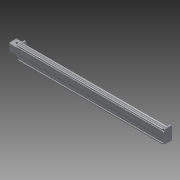
# Autodesk Inventor part: GL15N21240NSW' Body2
Saved by Autodesk Inventor 2011 SP1 (Build 150282100, 282)
## iProperties
Created: 2013-10-23
Part Number: GL15N21240NSW' Body2
Catalog Web Link: www.cadenas.de
Description: Type GL-N-body2-
Vendor: THK
Document SubType Name: Modeling
Designer: PARTuser1
Manufacturer: THK
Density: 1 g/cm^3
Category: PARTsolutions
Company: THK
Title: GL15N21240NSW' Body2
Author: Cadenas PARTsolutions
PSOL_IDENT_0: {$CADENAS_DATA\23d-libs\thk\actuator\type_gl_n\type_gl_n_f_na_1.prj},213 {VTYP=3D},{NB=GL15N21240NSW
PSOL_IDENT_1: ' Body2},{LINA=GL15N21240NSW' Body2},{NN=Type GL-N-body2},{DATE=29.11.2012 11:43:39},{GEOMDATE=29.11
PSOL_IDENT_2: .2012 11:43:00},{VERSION=},{LINEID=20},{LINESUBID=-1},{WBVAR=L,C,LM,BSE,BSM,LML,BSL}  {NB=GL15N21240
PSOL_IDENT_3: NSW' Body2},{LINA=GL15N21240NSW' Body2},{KT=DUMMY},{IDNR=},{MN=GL15N},{L=1240},{C=N},{LX=340,460,580
PSOL_IDENT_4: ,700,820,1060,1240,1420,1600,1780,1960},{LM=SW},{VER=2},{DS=Belt kit},{BSE=},{R=25.000},{NDM=2.000},
PSOL_IDENT_5: {PCD=0.000},{BSM=},{BSE1='','None'},{SD=39},{SD1=27},{TL=154.000},{B=52.000},{TL1=180.000},{B1=55.00
PSOL_IDENT_6: 0},{DS1=Ex},{LML='},{BSL=},{BSL1='','None'},{N=7},{N1=5},{N2=7.000},{N3=5},{BSM1='','None'}
CNS_NB: GL15N21240NSW' Body2
CNS_NBSYN: $MN.$VER.$L.$C.$BSE.$BSM.$LM.$LML.$BSL. Body2
CNS_LINA: GL15N21240NSW' Body2
CNS_MN: GL15N
CNS_L: 1240
CNS_C: No
CNS_LX: 340,460,580,700,820,1060,1240,1420,1600,1780,1960
CNS_LM: SSR-XW (L-type table)
CNS_VER: 2
CNS_DS: Belt kit
CNS_R: 25.000
CNS_NDM: 2.000
CNS_PCD: 0.000
CNS_BSE1: '','None'
CNS_SD: 39
CNS_SD1: 27
CNS_TL: 154.000
CNS_B: 52.000
CNS_TL1: 180.000
CNS_B1: 55.000
CNS_DS1: Ex
CNS_LML: No mark:Not provided with QZ
CNS_BSL1: '','None'
CNS_N: 7.000
CNS_N1: 5.000
CNS_N2: 7.000
CNS_N3: 5.000
CNS_BSM1: '','None'
SUPPLIER: THK
ARTICLENO: GL15N21240NSW' Body2
BOMINFO: GL15N21240NSW' Body2
CREATOR: CADENAS GmbH
Autodesk Inventor part; units mm, degrees
sketch "Sketch_1" plane through (0, 0, 0) normal (1, 0, 0) x (0, 1, 0)
  line L0 (18.1, 58) -> (12.47, 58)
  arc A0 (12.47, 58) -> (12, 57.53) centre (12.47, 57.53) ccw
  line L1 (12, 57.53) -> (12, 54.97)
  arc A1 (11.53, 54.5) -> (12, 54.97) centre (11.53, 54.97) ccw
  line L2 (11.53, 54.5) -> (6.47, 54.5)
  arc A2 (6, 54.97) -> (6.47, 54.5) centre (6.47, 54.97) ccw
  line L3 (6, 54.97) -> (6, 57.53)
  arc A3 (6, 57.53) -> (5.53, 58) centre (5.53, 57.53) ccw
  line L4 (5.53, 58) -> (3.14, 58)
  arc A4 (3.14, 58) -> (0, 54.86) centre (3.14, 54.86) ccw
  line L5 (0, 54.86) -> (0, 48.5)
  arc A5 (0, 48.5) -> (0.5, 48) centre (0.5, 48.5) ccw
  line L6 (0.5, 48) -> (3.5, 48)
  arc A6 (3.5, 48) -> (4, 48.5) centre (3.5, 48.5) ccw
  line L7 (4, 48.5) -> (4, 50)
  arc A7 (4.5, 50.5) -> (4, 50) centre (4.5, 50) ccw
  line L8 (4.5, 50.5) -> (8.5, 50.5)
  arc A8 (9, 50) -> (8.5, 50.5) centre (8.5, 50) ccw
  line L9 (9, 50) -> (9, 48.8)
  arc A9 (9, 48.8) -> (9.3, 48.5) centre (9.3, 48.8) ccw
  line L10 (9.3, 48.5) -> (9.7, 48.5)
  arc A10 (10, 48.2) -> (9.7, 48.5) centre (9.7, 48.2) ccw
  line L11 (10, 48.2) -> (10, 41.8)
  arc A11 (9.7, 41.5) -> (10, 41.8) centre (9.7, 41.8) ccw
  line L12 (9.7, 41.5) -> (9.3, 41.5)
  arc A12 (9.3, 41.5) -> (9, 41.2) centre (9.3, 41.2) ccw
  line L13 (9, 41.2) -> (9, 40)
  arc A13 (8.5, 39.5) -> (9, 40) centre (8.5, 40) ccw
  line L14 (8.5, 39.5) -> (4.5, 39.5)
  arc A14 (4, 40) -> (4.5, 39.5) centre (4.5, 40) ccw
  line L15 (4, 40) -> (4, 41.5)
  arc A15 (4, 41.5) -> (3.5, 42) centre (3.5, 41.5) ccw
  line L16 (3.5, 42) -> (0.5, 42)
  arc A16 (0.5, 42) -> (0, 41.5) centre (0.5, 41.5) ccw
  line L17 (0, 41.5) -> (0, 24)
  line L18 (0, 24) -> (0.531, 22.938)
  arc A17 (0.635, 22.4347) -> (0.531, 22.938) centre (-0.3634, 22.4908) ccw
  arc A18 (0.635, 22.4347) -> (0.635, -22.4347) centre (400.0054, 0) ccw
  arc A19 (0.531, -22.938) -> (0.635, -22.4347) centre (-0.3634, -22.4908) ccw
  line L19 (0.531, -22.938) -> (0, -24)
  line L20 (0, -24) -> (0, -41.5)
  arc A20 (0, -41.5) -> (0.5, -42) centre (0.5, -41.5) ccw
  line L21 (0.5, -42) -> (3.5, -42)
  arc A21 (3.5, -42) -> (4, -41.5) centre (3.5, -41.5) ccw
  line L22 (4, -41.5) -> (4, -40)
  arc A22 (4.5, -39.5) -> (4, -40) centre (4.5, -40) ccw
  line L23 (4.5, -39.5) -> (8.5, -39.5)
  arc A23 (9, -40) -> (8.5, -39.5) centre (8.5, -40) ccw
  line L24 (9, -40) -> (9, -41.2)
  arc A24 (9, -41.2) -> (9.3, -41.5) centre (9.3, -41.2) ccw
  line L25 (9.3, -41.5) -> (9.7, -41.5)
  arc A25 (10, -41.8) -> (9.7, -41.5) centre (9.7, -41.8) ccw
  line L26 (10, -41.8) -> (10, -48.2)
  arc A26 (9.7, -48.5) -> (10, -48.2) centre (9.7, -48.2) ccw
  line L27 (9.7, -48.5) -> (9.3, -48.5)
  arc A27 (9.3, -48.5) -> (9, -48.8) centre (9.3, -48.8) ccw
  line L28 (9, -48.8) -> (9, -50)
  arc A28 (8.5, -50.5) -> (9, -50) centre (8.5, -50) ccw
  line L29 (8.5, -50.5) -> (4.5, -50.5)
  arc A29 (4, -50) -> (4.5, -50.5) centre (4.5, -50) ccw
  line L30 (4, -50) -> (4, -48.5)
  arc A30 (4, -48.5) -> (3.5, -48) centre (3.5, -48.5) ccw
  line L31 (3.5, -48) -> (0.5, -48)
  arc A31 (0.5, -48) -> (0, -48.5) centre (0.5, -48.5) ccw
  line L32 (0, -48.5) -> (0, -54.86)
  arc A32 (0, -54.86) -> (3.14, -58) centre (3.14, -54.86) ccw
  line L33 (3.14, -58) -> (5.53, -58)
  arc A33 (5.53, -58) -> (6, -57.53) centre (5.53, -57.53) ccw
  line L34 (6, -57.53) -> (6, -54.97)
  arc A34 (6.47, -54.5) -> (6, -54.97) centre (6.47, -54.97) ccw
  line L35 (6.47, -54.5) -> (11.53, -54.5)
  arc A35 (12, -54.97) -> (11.53, -54.5) centre (11.53, -54.97) ccw
  line L36 (12, -54.97) -> (12, -57.53)
  arc A36 (12, -57.53) -> (12.47, -58) centre (12.47, -57.53) ccw
  line L37 (12.47, -58) -> (18.1, -58)
  line L38 (18.1, -58) -> (18.1, -57)
  line L39 (18.1, -57) -> (20.98, -57)
  arc A37 (20.98, -57) -> (21.45, -56.53) centre (20.98, -56.53) ccw
  line L40 (21.45, -56.53) -> (21.45, -55.97)
  arc A38 (21.45, -55.97) -> (20.98, -55.5) centre (20.98, -55.97) ccw
  line L41 (20.98, -55.5) -> (20.9, -55.5)
  arc A39 (20.7, -55.3) -> (20.9, -55.5) centre (20.9, -55.3) ccw
  line L42 (20.7, -55.3) -> (20.7, -53.3)
  arc A40 (21, -53) -> (20.7, -53.3) centre (21, -53.3) ccw
  line L43 (21, -53) -> (22, -53)
  arc A41 (22, -53) -> (22.2, -52.8) centre (22, -52.8) ccw
  arc A42 (22.5, -52.5) -> (22.2, -52.8) centre (22.5, -52.8) ccw
  line L44 (22.5, -52.5) -> (24.7, -52.5)
  arc A43 (25, -52.8) -> (24.7, -52.5) centre (24.7, -52.8) ccw
  arc A44 (25, -52.8) -> (25.2, -53) centre (25.2, -52.8) ccw
  line L45 (25.2, -53) -> (26.2, -53)
  arc A45 (26.5, -53.3) -> (26.2, -53) centre (26.2, -53.3) ccw
  line L46 (26.5, -53.3) -> (26.5, -55.3)
  arc A46 (26.3, -55.5) -> (26.5, -55.3) centre (26.3, -55.3) ccw
  line L47 (26.3, -55.5) -> (26.22, -55.5)
  arc A47 (26.22, -55.5) -> (25.75, -55.97) centre (26.22, -55.97) ccw
  line L48 (25.75, -55.97) -> (25.75, -56.53)
  arc A48 (25.75, -56.53) -> (26.22, -57) centre (26.22, -56.53) ccw
  line L49 (26.22, -57) -> (29.1, -57)
  line L50 (29.1, -57) -> (29.1, -58)
  line L51 (29.1, -58) -> (31.6, -58)
  line L52 (31.6, -58) -> (33, -56.6)
  line L53 (33, -56.6) -> (33, -52.5)
  line L54 (33, -52.5) -> (34.32, -52.5)
  line L55 (34.32, -52.5) -> (37.42, -49.4)
  line L56 (37.42, -49.4) -> (40.4, -49.4)
  line L57 (40.4, -49.4) -> (43.5, -52.5)
  line L58 (43.5, -52.5) -> (44.8, -52.5)
  line L59 (44.8, -52.5) -> (45.6, -51.7)
  line L60 (45.6, -51.7) -> (45.6, -38.3)
  line L61 (45.6, -38.3) -> (44.8, -37.5)
  line L62 (44.8, -37.5) -> (43.5, -37.5)
  line L63 (43.5, -37.5) -> (40.37, -40.63)
  line L64 (40.37, -40.63) -> (37.45, -40.63)
  line L65 (37.45, -40.63) -> (34.32, -37.5)
  line L66 (34.32, -37.5) -> (32.2, -37.5)
  line L67 (32.2, -37.5) -> (32.2, -33.5)
  arc A49 (32.2, -33.5) -> (31.7, -33) centre (31.7, -33.5) ccw
  line L68 (31.7, -33) -> (17, -33)
  arc A50 (16, -32) -> (17, -33) centre (17, -32) ccw
  line L69 (16, -32) -> (16, 32)
  arc A51 (17, 33) -> (16, 32) centre (17, 32) ccw
  line L70 (17, 33) -> (31.7, 33)
  arc A52 (31.7, 33) -> (32.2, 33.5) centre (31.7, 33.5) ccw
  line L71 (32.2, 33.5) -> (32.2, 37.5)
  line L72 (32.2, 37.5) -> (34.32, 37.5)
  line L73 (34.32, 37.5) -> (37.45, 40.63)
  line L74 (37.45, 40.63) -> (40.37, 40.63)
  line L75 (40.37, 40.63) -> (43.5, 37.5)
  line L76 (43.5, 37.5) -> (44.8, 37.5)
  line L77 (44.8, 37.5) -> (45.6, 38.3)
  line L78 (45.6, 38.3) -> (45.6, 51.7)
  line L79 (45.6, 51.7) -> (44.8, 52.5)
  line L80 (44.8, 52.5) -> (43.5, 52.5)
  line L81 (43.5, 52.5) -> (40.4, 49.4)
  line L82 (40.4, 49.4) -> (37.42, 49.4)
  line L83 (37.42, 49.4) -> (34.32, 52.5)
  line L84 (34.32, 52.5) -> (33, 52.5)
  line L85 (33, 52.5) -> (33, 56.6)
  line L86 (33, 56.6) -> (31.6, 58)
  line L87 (31.6, 58) -> (29.1, 58)
  line L88 (29.1, 58) -> (29.1, 57)
  line L89 (29.1, 57) -> (26.22, 57)
  arc A53 (26.22, 57) -> (25.75, 56.53) centre (26.22, 56.53) ccw
  line L90 (25.75, 56.53) -> (25.75, 55.97)
  arc A54 (25.75, 55.97) -> (26.22, 55.5) centre (26.22, 55.97) ccw
  line L91 (26.22, 55.5) -> (26.3, 55.5)
  arc A55 (26.5, 55.3) -> (26.3, 55.5) centre (26.3, 55.3) ccw
  line L92 (26.5, 55.3) -> (26.5, 53.3)
  arc A56 (26.2, 53) -> (26.5, 53.3) centre (26.2, 53.3) ccw
  line L93 (26.2, 53) -> (25.2, 53)
  arc A57 (25.2, 53) -> (25, 52.8) centre (25.2, 52.8) ccw
  arc A58 (24.7, 52.5) -> (25, 52.8) centre (24.7, 52.8) ccw
  line L94 (24.7, 52.5) -> (22.5, 52.5)
  arc A59 (22.2, 52.8) -> (22.5, 52.5) centre (22.5, 52.8) ccw
  arc A60 (22.2, 52.8) -> (22, 53) centre (22, 52.8) ccw
  line L95 (22, 53) -> (21, 53)
  arc A61 (20.7, 53.3) -> (21, 53) centre (21, 53.3) ccw
  line L96 (20.7, 53.3) -> (20.7, 55.3)
  arc A62 (20.9, 55.5) -> (20.7, 55.3) centre (20.9, 55.3) ccw
  line L97 (20.9, 55.5) -> (20.98, 55.5)
  arc A63 (20.98, 55.5) -> (21.45, 55.97) centre (20.98, 55.97) ccw
  line L98 (21.45, 55.97) -> (21.45, 56.53)
  arc A64 (21.45, 56.53) -> (20.98, 57) centre (20.98, 56.53) ccw
  line L99 (20.98, 57) -> (18.1, 57)
  line L100 (18.1, 57) -> (18.1, 58)
  constraints: 202 end point, 130 point on circle, 65 centre point
extrude "Extrusion1" add sketch "Sketch_1" along normal blind 1240
sketch "Sketch_2" plane through (0, 0, 0) normal (1, 0, 0) x (0, 1, 0)
  line L0 (68.3, 57) -> (27.6, 57)
  line L1 (27.6, 57) -> (27.6, 53)
  line L2 (27.6, 53) -> (19.6, 53)
  line L3 (19.6, 53) -> (19.6, 57)
  line L4 (19.6, 57) -> (12.12, 57)
  line L5 (12.12, 57) -> (10, 54.88)
  line L6 (10, 54.88) -> (10, 38.5)
  line L7 (10, 38.5) -> (3.41, 38.5)
  line L8 (3.41, 38.5) -> (2, 37.09)
  line L9 (2, 37.09) -> (2, -37.09)
  line L10 (2, -37.09) -> (3.41, -38.5)
  line L11 (3.41, -38.5) -> (10, -38.5)
  line L12 (10, -38.5) -> (10, -54.88)
  line L13 (10, -54.88) -> (12.12, -57)
  line L14 (12.12, -57) -> (19.6, -57)
  line L15 (19.6, -57) -> (19.6, -53)
  line L16 (19.6, -53) -> (27.6, -53)
  line L17 (27.6, -53) -> (27.6, -57)
  line L18 (27.6, -57) -> (68.3, -57)
  line L19 (68.3, -57) -> (68.3, -50)
  line L20 (68.3, -50) -> (72.3, -50)
  line L21 (72.3, -50) -> (72.3, 50)
  line L22 (72.3, 50) -> (68.3, 50)
  line L23 (68.3, 50) -> (68.3, 57)
  constraints: 48 end point
extrude "Extrusion2" add sketch "Sketch_2" against normal blind 12
sketch "Sketch_3" plane through (1240, 0, 0) normal (1, 0, 0) x (0, 0, -1)
  line L0 (-57, 68.3) -> (-57, 27.6)
  line L1 (-57, 27.6) -> (-53, 27.6)
  line L2 (-53, 27.6) -> (-53, 19.6)
  line L3 (-53, 19.6) -> (-57, 19.6)
  line L4 (-57, 19.6) -> (-57, 12.12)
  line L5 (-57, 12.12) -> (-54.88, 10)
  line L6 (-54.88, 10) -> (-38.5, 10)
  line L7 (-38.5, 10) -> (-38.5, 3.41)
  line L8 (-38.5, 3.41) -> (-37.09, 2)
  line L9 (-37.09, 2) -> (37.09, 2)
  line L10 (37.09, 2) -> (38.5, 3.41)
  line L11 (38.5, 3.41) -> (38.5, 10)
  line L12 (38.5, 10) -> (54.88, 10)
  line L13 (54.88, 10) -> (57, 12.12)
  line L14 (57, 12.12) -> (57, 19.6)
  line L15 (57, 19.6) -> (53, 19.6)
  line L16 (53, 19.6) -> (53, 27.6)
  line L17 (53, 27.6) -> (57, 27.6)
  line L18 (57, 27.6) -> (57, 68.3)
  line L19 (57, 68.3) -> (50, 68.3)
  line L20 (50, 68.3) -> (50, 72.3)
  line L21 (50, 72.3) -> (-50, 72.3)
  line L22 (-50, 72.3) -> (-50, 68.3)
  line L23 (-50, 68.3) -> (-57, 68.3)
  constraints: 48 end point
extrude "Extrusion3" add sketch "Sketch_3" along normal blind 12
sketch "Sketch4" plane through (0, 72.3, 50) normal (0, 1, 0) x (1, 0, 0)
  point P0 (-6, 82)
hole "Drilling 1" at (-6, 72.3, -32) direction (0, -1, 0) diameter 2.459 depth 5.5 tip angle 120.691 countersink diameter 3 countersink angle 90 thread size "M3x0.5" class "6H" standard "ISO Metric profile"
sketch "Sketch5" plane through (0, 72.3, 50) normal (0, 1, 0) x (1, 0, 0)
  point P0 (-6, 18)
hole "Drilling 2" at (-6, 72.3, 32) direction (0, -1, 0) diameter 2.459 depth 5.5 tip angle 120.691 countersink diameter 3 countersink angle 90 thread size "M3x0.5" class "6H" standard "ISO Metric profile"
sketch "Sketch6" plane through (1240, 72.3, 50) normal (0, 1, 0) x (1, 0, 0)
  point P0 (6, 82)
hole "Drilling 3" at (1246, 72.3, -32) direction (0, -1, 0) diameter 2.459 depth 5.5 tip angle 120.691 countersink diameter 3 countersink angle 90 thread size "M3x0.5" class "6H" standard "ISO Metric profile"
sketch "Sketch7" plane through (1240, 72.3, 50) normal (0, 1, 0) x (1, 0, 0)
  point P0 (6, 18)
hole "Drilling 4" at (1246, 72.3, 32) direction (0, -1, 0) diameter 2.459 depth 5.5 tip angle 120.691 countersink diameter 3 countersink angle 90 thread size "M3x0.5" class "6H" standard "ISO Metric profile"
sketch "Sketch8" plane through (1252, 0, 0) normal (1, 0, 0) x (0, 0, -1)
  point P0 (38, 64.5)
hole "Drilling 5" at (1252, 64.5, -38) direction (-1, 0, 0) diameter 4.134 depth 12 countersink diameter 5 countersink angle 90 thread size "M5x0.8" class "6H" standard "ISO Metric profile"
sketch "Sketch_5" plane through (0, 0, 0) normal (1, 0, 0) x (0, 1, 0)
  line L0 (66.8094, -34) -> (62.1906, -34)
  line L1 (62.1906, -34) -> (59.8812, -38)
  line L2 (59.8812, -38) -> (62.1906, -42)
  line L3 (62.1906, -42) -> (66.8094, -42)
  line L4 (66.8094, -42) -> (69.1188, -38)
  line L5 (69.1188, -38) -> (66.8094, -34)
  constraints: 12 end point
extrude "Extrusion4" add sketch "Sketch_5" along normal blind 3.2
sketch "Sketch_6" plane through (0, 0, -38) normal (0, 0, 1) x (1, 0, 0)
  line L0 (15, 64.5) -> (3.2, 64.5)
  line L1 (3.2, 64.5) -> (3.2, 67)
  line L2 (3.2, 67) -> (6, 67)
  line L3 (6, 67) -> (6, 70.75)
  line L4 (6, 70.75) -> (15, 70.75)
  line L5 (15, 70.75) -> (15, 64.5)
  line L6 (15, 64.5) -> (3.2, 64.5)
  constraints: 14 end point
revolve "Revolution1" add sketch "Sketch_6" angle 360 about axis through (15, 64.5, -38) along (1, 0, 0)
sketch "Sketch_7" plane through (1237.5, 0, 0) normal (1, 0, 0) x (0, 0, -1)
  line L0 (-29, 16) -> (29, 16)
  line L1 (29, 16) -> (29, 30.5)
  line L2 (29, 30.5) -> (-29, 30.5)
  line L3 (-29, 30.5) -> (-29, 16)
  constraints: 8 end point
extrude "Extrusion5" add sketch "Sketch_7" against normal blind 63
sketch "Sketch_8" plane through (0, 30.5, 0) normal (0, 1, 0) x (1, 0, 0)
  line L0 (1142, -29) -> (1223, -29)
  line L1 (1223, -29) -> (1223, 29)
  line L2 (1223, 29) -> (1142, 29)
  line L3 (1142, 29) -> (1142, 17)
  line L4 (1142, 17) -> (1177, 17)
  line L5 (1177, 17) -> (1177, -17)
  line L6 (1177, -17) -> (1142, -17)
  line L7 (1142, -17) -> (1142, -29)
  arc A0 (1182, -20.4) -> (1182, -25.6) centre (1182, -23) ccw
  line L8 (1182, -25.6) -> (1216, -25.6)
  arc A1 (1216, -25.6) -> (1216, -20.4) centre (1216, -23) ccw
  line L9 (1216, -20.4) -> (1182, -20.4)
  arc A2 (1182, 25.6) -> (1182, 20.4) centre (1182, 23) ccw
  line L10 (1182, 20.4) -> (1216, 20.4)
  arc A3 (1216, 20.4) -> (1216, 25.6) centre (1216, 23) ccw
  line L11 (1216, 25.6) -> (1182, 25.6)
  constraints: 24 end point, 8 point on circle, 4 centre point
extrude "Extrusion6" add sketch "Sketch_8" along normal blind 20
sketch "Sketch_9" plane through (0, 0, 0) normal (0, 0, 1) x (1, 0, 0)
  line L0 (-86, 69.3) -> (-86, 11.7)
  line L1 (-86, 11.7) -> (-81.8, 7.5)
  line L2 (-81.8, 7.5) -> (-12, 7.5)
  line L3 (-12, 7.5) -> (-12, 73.5)
  line L4 (-12, 73.5) -> (-81.8, 73.5)
  line L5 (-81.8, 73.5) -> (-86, 69.3)
  constraints: 12 end point
extrude "Extrusion7" add sketch "Sketch_9" along normal mid plane 60
sketch "Sketch_14" plane through (0, 17.5, 0) normal (0, 1, 0) x (1, 0, 0)
  arc A0 (-49, 20) -> (-49, -20) centre (-49, 0) ccw
  line L0 (-49, -20) -> (0, -20)
  line L1 (0, -20) -> (0, 20)
  line L2 (0, 20) -> (-49, 20)
  constraints: 6 end point, 2 point on circle, 1 centre point
extrude "Extrusion8" cut sketch "Sketch_14" along normal blind 46
sketch "Sketch_15" plane through (1152, 0, 0) normal (1, 0, 0) x (0, 0, -1)
  line L0 (31.15, 40.5) -> (-31.15, 40.5)
  line L1 (-31.15, 40.5) -> (-31.15, 45.5)
  line L2 (-31.15, 45.5) -> (-15.3, 45.5)
  line L3 (-15.3, 45.5) -> (-15.3, 60)
  line L4 (-15.3, 60) -> (-13.8, 60)
  line L5 (-13.8, 60) -> (-13.3, 58.05)
  line L6 (-13.3, 58.05) -> (13.3, 58.05)
  line L7 (13.3, 58.05) -> (13.8, 60)
  line L8 (13.8, 60) -> (15.3, 60)
  line L9 (15.3, 60) -> (15.3, 45.5)
  line L10 (15.3, 45.5) -> (31.15, 45.5)
  line L11 (31.15, 45.5) -> (31.15, 40.5)
  line L12 (31.15, 40.5) -> (-31.15, 40.5)
  constraints: 26 end point
revolve "Revolution2" add sketch "Sketch_15" angle 360 about axis through (1152, 40.5, -31.15) along (0, 0, -1)
sketch "Sketch_16" plane through (0, 0, 30) normal (0, 0, 1) x (1, 0, 0)
  circle A0 centre (-49, 40.5) radius 10
  constraints: 1 centre point
extrude "Extrusion9" cut sketch "Sketch_16" along normal mid plane 5
sketch "Sketch17" plane through (0, 0, -30) normal (0, 0, -1) x (-1, 0, 0)
  point P0 (49, 40.5)
hole "Drilling 7" at (-49, 40.5, -30) direction (0, 0, 1) diameter 20 depth 2.5
sketch "Sketch_18" plane through (-49, 0, 0) normal (1, 0, 0) x (0, 0, -1)
  line L0 (28, 40.5) -> (-42, 40.5)
  line L1 (-42, 40.5) -> (-42, 45)
  line L2 (-42, 45) -> (-41.5, 45.5)
  line L3 (-41.5, 45.5) -> (-15.3, 45.5)
  line L4 (-15.3, 45.5) -> (-15.3, 60)
  line L5 (-15.3, 60) -> (-13.8, 60)
  line L6 (-13.8, 60) -> (-13.3, 58.05)
  line L7 (-13.3, 58.05) -> (13.3, 58.05)
  line L8 (13.3, 58.05) -> (13.8, 60)
  line L9 (13.8, 60) -> (15.3, 60)
  line L10 (15.3, 60) -> (15.3, 45.5)
  line L11 (15.3, 45.5) -> (28, 45.5)
  line L12 (28, 45.5) -> (28, 40.5)
  line L13 (28, 40.5) -> (-42, 40.5)
  constraints: 28 end point
revolve "Revolution3" add sketch "Sketch_18" angle 360 about axis through (-49, 40.5, -28) along (0, 0, -1)
sketch "Sketch_19" plane through (0, 0, 0) normal (0, 0, 1) x (1, 0, 0)
  arc A0 (-49, 59) -> (-49, 22) centre (-49, 40.5) ccw
  line L0 (-49, 22) -> (1152, 22)
  arc A1 (1152, 22) -> (1152, 59) centre (1152, 40.5) ccw
  line L1 (1152, 59) -> (-49, 59)
  arc A2 (-49, 55.8) -> (-49, 25.2) centre (-49, 40.5) ccw
  line L2 (-49, 25.2) -> (1152, 25.2)
  arc A3 (1152, 25.2) -> (1152, 55.8) centre (1152, 40.5) ccw
  line L3 (1152, 55.8) -> (-49, 55.8)
  constraints: 8 end point, 8 point on circle, 4 centre point
extrude "Extrusion10" add sketch "Sketch_19" along normal mid plane 25
sketch "Sketch_20" plane through (1229.5, 0, 0) normal (1, 0, 0) x (0, 0, -1)
  line L0 (23, 30.5) -> (23, 37.5)
  line L1 (23, 37.5) -> (28, 37.5)
  line L2 (28, 37.5) -> (28, 31.5)
  line L3 (28, 31.5) -> (28.5, 31.5)
  line L4 (28.5, 31.5) -> (28.5, 30.5)
  line L5 (28.5, 30.5) -> (23, 30.5)
  line L6 (23, 30.5) -> (23, 37.5)
  constraints: 14 end point
revolve "Revolution4" add sketch "Sketch_20" angle 360 about axis through (1229.5, 30.5, -23) along (0, -1, 0)
sketch "Sketch_21" plane through (1229.5, 0, 0) normal (1, 0, 0) x (0, 0, -1)
  line L0 (-23, 30.5) -> (-23, 37.5)
  line L1 (-23, 37.5) -> (-18, 37.5)
  line L2 (-18, 37.5) -> (-18, 31.5)
  line L3 (-18, 31.5) -> (-17.5, 31.5)
  line L4 (-17.5, 31.5) -> (-17.5, 30.5)
  line L5 (-17.5, 30.5) -> (-23, 30.5)
  line L6 (-23, 30.5) -> (-23, 37.5)
  constraints: 14 end point
revolve "Revolution5" add sketch "Sketch_21" angle 360 about axis through (1229.5, 30.5, 23) along (0, -1, 0)
sketch "Sketch_22" plane through (1216, 0, 0) normal (1, 0, 0) x (0, 0, -1)
  line L0 (23, 50.5) -> (23, 56.5)
  line L1 (23, 56.5) -> (27.25, 56.5)
  line L2 (27.25, 56.5) -> (27.25, 51.5)
  line L3 (27.25, 51.5) -> (28, 51.5)
  line L4 (28, 51.5) -> (28, 50.5)
  line L5 (28, 50.5) -> (23, 50.5)
  line L6 (23, 50.5) -> (23, 56.5)
  constraints: 14 end point
revolve "Revolution6" add sketch "Sketch_22" angle 360 about axis through (1216, 50.5, -23) along (0, -1, 0)
sketch "Sketch_23" plane through (1216, 0, 0) normal (1, 0, 0) x (0, 0, -1)
  line L0 (-23, 50.5) -> (-23, 56.5)
  line L1 (-23, 56.5) -> (-18.75, 56.5)
  line L2 (-18.75, 56.5) -> (-18.75, 51.5)
  line L3 (-18.75, 51.5) -> (-18, 51.5)
  line L4 (-18, 51.5) -> (-18, 50.5)
  line L5 (-18, 50.5) -> (-23, 50.5)
  line L6 (-23, 50.5) -> (-23, 56.5)
  constraints: 14 end point
revolve "Revolution7" add sketch "Sketch_23" angle 360 about axis through (1216, 50.5, 23) along (0, -1, 0)
sketch "Sketch_24" plane through (1196, 0, 0) normal (1, 0, 0) x (0, 0, -1)
  line L0 (23, 50.5) -> (23, 56.5)
  line L1 (23, 56.5) -> (27.25, 56.5)
  line L2 (27.25, 56.5) -> (27.25, 51.5)
  line L3 (27.25, 51.5) -> (28, 51.5)
  line L4 (28, 51.5) -> (28, 50.5)
  line L5 (28, 50.5) -> (23, 50.5)
  line L6 (23, 50.5) -> (23, 56.5)
  constraints: 14 end point
revolve "Revolution8" add sketch "Sketch_24" angle 360 about axis through (1196, 50.5, -23) along (0, -1, 0)
sketch "Sketch_25" plane through (1196, 0, 0) normal (1, 0, 0) x (0, 0, -1)
  line L0 (-23, 50.5) -> (-23, 56.5)
  line L1 (-23, 56.5) -> (-18.75, 56.5)
  line L2 (-18.75, 56.5) -> (-18.75, 51.5)
  line L3 (-18.75, 51.5) -> (-18, 51.5)
  line L4 (-18, 51.5) -> (-18, 50.5)
  line L5 (-18, 50.5) -> (-23, 50.5)
  line L6 (-23, 50.5) -> (-23, 56.5)
  constraints: 14 end point
revolve "Revolution9" add sketch "Sketch_25" angle 360 about axis through (1196, 50.5, 23) along (0, -1, 0)
sketch "Sketch26" plane through (0, 0, 30) normal (0, 0, 1) x (1, 0, 0)
  point P0 (-22.1299, 13.6299)
hole "Drilling 8" at (-22.1299, 13.6299, 30) direction (0, 0, -1) diameter 4.134 depth 9.6 tip angle 119.725 countersink diameter 5 countersink angle 90 thread size "M5x0.8" class "6H" standard "ISO Metric profile"
sketch "Sketch27" plane through (0, 0, 30) normal (0, 0, 1) x (1, 0, 0)
  point P0 (-75.8701, 67.3701)
hole "Drilling 9" at (-75.8701, 67.3701, 30) direction (0, 0, -1) diameter 4.134 depth 9.6 tip angle 119.725 countersink diameter 5 countersink angle 90 thread size "M5x0.8" class "6H" standard "ISO Metric profile"
sketch "Sketch28" plane through (0, 0, 30) normal (0, 0, 1) x (1, 0, 0)
  point P0 (-22.1299, 67.3701)
hole "Drilling 10" at (-22.1299, 67.3701, 30) direction (0, 0, -1) diameter 4.134 depth 9.6 tip angle 119.725 countersink diameter 5 countersink angle 90 thread size "M5x0.8" class "6H" standard "ISO Metric profile"
sketch "Sketch29" plane through (0, 0, 30) normal (0, 0, 1) x (1, 0, 0)
  point P0 (-75.8701, 13.6299)
hole "Drilling 11" at (-75.8701, 13.6299, 30) direction (0, 0, -1) diameter 4.134 depth 9.6 tip angle 119.725 countersink diameter 5 countersink angle 90 thread size "M5x0.8" class "6H" standard "ISO Metric profile"
sketch "Sketch30" plane through (0, 16, 32) normal (0, 1, 0) x (1, 0, 0)
  point P0 (30, 7)
hole "Drilling 12" at (30, 16, 25) direction (0, -1, 0) diameter 6.6 depth 16 counterbore diameter 11 counterbore depth 11
pattern_linear "Rectangular Pattern1" count 8 spacing 150 along (1, 0, 0) of "Drilling 12"
sketch "Sketch31" plane through (0, 16, 32) normal (0, 1, 0) x (1, 0, 0)
  point P0 (30, 57)
hole "Drilling 13" at (30, 16, -25) direction (0, -1, 0) diameter 6.6 depth 16 counterbore diameter 11 counterbore depth 11
pattern_linear "Rectangular Pattern2" count 8 spacing 150 along (1, 0, 0) of "Drilling 13"
ref_plane "type_gl_n_bt_XY" through (15, 38, 0) normal (-1, 0, 0) x (0, 0, -1)
ref_plane "type_gl_n_bt_YZ" through (15, 38, 0) normal (0, 0, -1) x (0, -1, 0)
ref_plane "type_gl_n_bt_ZX" through (15, 38, 0) normal (0, -1, 0) x (-1, 0, 0)
ref_plane "type_gl_n_bx_XY" through (-49, 40.5, 30) normal (0, 0, -1) x (1, 0, 0)
ref_plane "type_gl_n_bx_YZ" through (-49, 40.5, 30) normal (1, 0, 0) x (0, -1, 0)
ref_plane "type_gl_n_bx_ZX" through (-49, 40.5, 30) normal (0, -1, 0) x (0, 0, -1)
ref_plane "type_gl_n_dummy1_XY" through (0, 0, 0) normal (0, 1, 0) x (1, 0, 0)
ref_plane "type_gl_n_dummy1_YZ" through (0, 0, 0) normal (1, 0, 0) x (0, 0, -1)
ref_plane "type_gl_n_dummy1_ZX" through (0, 0, 0) normal (0, 0, -1) x (0, 1, 0)
ref_plane "type_gl_n_s1_XY" through (47, 23.6, 53) normal (0, 0, -1) x (1, 0, 0)
ref_plane "type_gl_n_s1_YZ" through (47, 23.6, 53) normal (1, 0, 0) x (0, -1, 0)
ref_plane "type_gl_n_s1_ZX" through (47, 23.6, 53) normal (0, -1, 0) x (0, 0, -1)
ref_plane "type_gl_n_s2_XY" through (550.75, 23.6, 53) normal (0, 0, -1) x (1, 0, 0)
ref_plane "type_gl_n_s2_YZ" through (550.75, 23.6, 53) normal (1, 0, 0) x (0, -1, 0)
ref_plane "type_gl_n_s2_ZX" through (550.75, 23.6, 53) normal (0, -1, 0) x (0, 0, -1)
ref_plane "type_gl_n_s3_XY" through (1049, 23.6, 53) normal (0, 0, -1) x (1, 0, 0)
ref_plane "type_gl_n_s3_YZ" through (1049, 23.6, 53) normal (1, 0, 0) x (0, -1, 0)
ref_plane "type_gl_n_s3_ZX" through (1049, 23.6, 53) normal (0, -1, 0) x (0, 0, -1)
body "Solid1"
